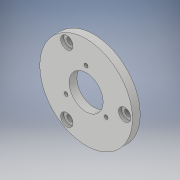
# Autodesk Inventor part: Encoder Mount Front
Saved by Autodesk Inventor 2018 (Build 220112000, 112)
## iProperties
Created: 2018-03-20
Part Number: Encoder Mount Front
Material: Generic
Document SubType Name: Modeling
Designer: P301319
Density: 1 g/cm^3
Appearance: Default
Author: P301319
Autodesk Inventor part; units mm, degrees
ref_plane "YZ Plane" through (0, 0, 0) normal (1, 0, 0) x (0, 1, 0)
ref_plane "XZ Plane" through (0, 0, 0) normal (0, 1, 0) x (-1, 0, 0)
ref_plane "XY Plane" through (0, 0, 0) normal (0, 0, 1) x (1, 0, 0)
sketch "Sketch1" plane through (0, 0, 0) normal (0, 0, 1) x (1, 0, 0)
  circle A0 centre (0, 0) radius 10
  circle A1 centre (0, 0) radius 30
  circle A2 centre (0, 15) radius 1.25
  circle A3 centre (-12.9904, -7.5) radius 1.25
  circle A4 centre (12.9904, -7.5) radius 1.25
  dimension "d0" = 20
  dimension "d1" = 60
  dimension "d3" = 2.5
  dimension "d6" = 360
  constraints: 5 centre point, 2 coincident, 7 other
  measures "d0" diameter of A0
  measures "d1" diameter of A1
  measures "d3" diameter of A2
extrude "Extrusion1" add sketch "Sketch1" along normal blind 5
sketch "Sketch2" plane through (0, 0, 5) normal (0, 0, 1) x (1, 0, 0)
  line L0 (0, 0) -> (25, 0) construction
  circle A0 centre (-12.5, -21.6506) radius 4
  circle A1 centre (0, 0) radius 10 projected
  circle A2 centre (25, 0) radius 4
  circle A3 centre (-12.5, 21.6506) radius 4
  dimension "d12" = 8
  dimension "d15" = 360
  constraints: 3 centre point, 2 end point, 1 horizontal, 7 other
  measures "d12" diameter of A0
extrude "Extrusion2" cut sketch "Sketch2" against normal blind 2 contours A3
extrude "Extrusion3" cut sketch "Sketch2" against normal blind 2 contours A0
extrude "Extrusion4" cut sketch "Sketch2" against normal blind 2 contours A2
sketch "Sketch3" plane through (-12.5, 21.6506, 3) normal (0, 0, 1) x (1, 0, 0)
  circle A0 centre (0, 0) radius 2
  circle A1 centre (0, -43.3013) radius 2
  circle A2 centre (37.5, -21.6506) radius 2
  point P0 (12.5, -21.6506)
  dimension "d23" = 4
  dimension "d26" = 360
  constraints: 3 centre point, 7 other
  measures "d23" diameter of A0
extrude "Extrusion5" cut sketch "Sketch3" against normal through all contours A0
extrude "Extrusion6" cut sketch "Sketch3" against normal through all contours A1
extrude "Extrusion7" cut sketch "Sketch3" against normal through all contours A2
sketch "Sketch4" plane through (0, 0, 5) normal (0, 0, 1) x (1, 0, 0)
  circle A0 centre (0, 0) radius 10 projected
  circle A1 centre (0, 0) radius 11
  dimension "d34" = 1
  constraints: 1 centre point
  measures "d34" radial gap between concentric circles of A0 A1
extrude "Extrusion8" cut sketch "Sketch4" against normal blind 10
body "Solid1"
